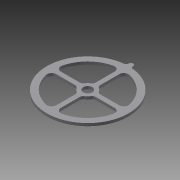
# Autodesk Inventor part: Vertical Thruster Grill 25090213
Saved by Autodesk Inventor 2013 (Build 170138000, 138)
## iProperties
Created: 2012-05-09
Part Number: Vertical Thruster Grill 25090213
Material: Generic
Document SubType Name: Modeling
Designer: user
Density: 1 g/cm^3
Author: user
Autodesk Inventor part; units mm, degrees
ref_plane "YZ Plane" through (0, 0, 0) normal (1, 0, 0) x (0, 1, 0)
ref_plane "XZ Plane" through (0, 0, 0) normal (0, 1, 0) x (-1, 0, 0)
ref_plane "XY Plane" through (0, 0, 0) normal (0, 0, 1) x (1, 0, 0)
sketch "Sketch1" plane through (0, 0, 0) normal (0, 0, 1) x (1, 0, 0)
  arc A0 (-4.7368, 44.75) -> (4.7368, 44.75) centre (0, 0) ccw
  line L0 (-32.2391, 2.5) -> (-11.2583, 2.5)
  line L1 (11.2583, 2.5) -> (32.2391, 2.5)
  line L2 (-2.5, 32.2391) -> (-2.5, 11.2583)
  line L3 (-2.5, -11.2583) -> (-2.5, -32.2391)
  line L4 (-32.2391, -2.5) -> (-11.2583, -2.5)
  line L5 (11.2583, -2.5) -> (32.2391, -2.5)
  line L6 (2.5, 32.2391) -> (2.5, 11.2583)
  line L7 (2.5, -11.2583) -> (2.5, -32.2391)
  arc A1 (-8.6329, 37.1091) -> (-37.1091, 8.6329) centre (0, 0) ccw
  arc A2 (37.1091, 8.6329) -> (8.6329, 37.1091) centre (0, 0) ccw
  arc A3 (-37.1091, -8.6329) -> (-8.6329, -37.1091) centre (0, 0) ccw
  arc A4 (8.6329, -37.1091) -> (37.1091, -8.6329) centre (0, 0) ccw
  arc A5 (-2.5, 32.2391) -> (-8.6329, 37.1091) centre (-7.5, 32.2391) ccw
  arc A6 (8.6329, 37.1091) -> (2.5, 32.2391) centre (7.5, 32.2391) ccw
  arc A7 (32.2391, 2.5) -> (37.1091, 8.6329) centre (32.2391, 7.5) ccw
  arc A8 (37.1091, -8.6329) -> (32.2391, -2.5) centre (32.2391, -7.5) ccw
  arc A9 (2.5, -32.2391) -> (8.6329, -37.1091) centre (7.5, -32.2391) ccw
  arc A10 (-8.6329, -37.1091) -> (-2.5, -32.2391) centre (-7.5, -32.2391) ccw
  arc A11 (-32.2391, -2.5) -> (-37.1091, -8.6329) centre (-32.2391, -7.5) ccw
  arc A12 (-37.1091, 8.6329) -> (-32.2391, 2.5) centre (-32.2391, 7.5) ccw
  line L8 (-2.5, 47.2361) -> (-2.5, 47.5)
  line L9 (0, 50) -> (0, 50)
  line L10 (2.5, 47.5) -> (2.5, 47.2361)
  arc A13 (0, 50) -> (-2.5, 47.5) centre (0, 47.5) ccw
  arc A14 (2.5, 47.5) -> (0, 50) centre (0, 47.5) ccw
  arc A15 (2.5, 47.2361) -> (4.7368, 44.75) centre (5, 47.2361) ccw
  arc A16 (-4.7368, 44.75) -> (-2.5, 47.2361) centre (-5, 47.2361) ccw
  circle A17 centre (0, 0) radius 5
  arc A18 (-4.5, 7.7942) -> (-7.7942, 4.5) centre (0, 0) ccw
  arc A19 (7.7942, 4.5) -> (4.5, 7.7942) centre (0, 0) ccw
  arc A20 (-7.7942, -4.5) -> (-4.5, -7.7942) centre (0, 0) ccw
  arc A21 (4.5, -7.7942) -> (7.7942, -4.5) centre (0, 0) ccw
  arc A22 (-11.2583, 2.5) -> (-7.7942, 4.5) centre (-11.2583, 6.5) ccw
  arc A23 (-4.5, 7.7942) -> (-2.5, 11.2583) centre (-6.5, 11.2583) ccw
  arc A24 (2.5, 11.2583) -> (4.5, 7.7942) centre (6.5, 11.2583) ccw
  arc A25 (7.7942, 4.5) -> (11.2583, 2.5) centre (11.2583, 6.5) ccw
  arc A26 (11.2583, -2.5) -> (7.7942, -4.5) centre (11.2583, -6.5) ccw
  arc A27 (4.5, -7.7942) -> (2.5, -11.2583) centre (6.5, -11.2583) ccw
  arc A28 (-2.5, -11.2583) -> (-4.5, -7.7942) centre (-6.5, -11.2583) ccw
  arc A29 (-7.7942, -4.5) -> (-11.2583, -2.5) centre (-11.2583, -6.5) ccw
  point P0 (-2.5, 38.0179)
  point P1 (2.5, 38.0179)
  point P2 (-38.0179, -2.5)
  point P3 (-38.0179, 2.5)
  point P4 (38.0179, -2.5)
  point P5 (38.0179, 2.5)
  point P6 (2.5, -38.0179)
  point P7 (-2.5, -38.0179)
  point P8 (-2.5, 44.9305)
  point P9 (2.5, 44.9305)
  point P10 (-2.5, 8.6458)
  point P11 (2.5, 8.6458)
  point P12 (8.6458, 2.5)
  point P13 (8.6458, -2.5)
  point P14 (2.5, -8.6458)
  point P15 (-2.5, -8.6458)
  point P16 (-8.6458, -2.5)
  point P17 (-8.6458, 2.5)
  dimension "d0" = 90
  dimension "d7" = 2.5
  dimension "d8" = 2.5
  dimension "d9" = 2.5
  dimension "d10" = 5
  dimension "d11" = 5
  dimension "d12" = 5
  dimension "d13" = 5
  dimension "d14" = 38.1
  dimension "d15" = 38.1
  dimension "d16" = 38.1
  dimension "d17" = 38.1
  dimension "d18" = 5
  dimension "d19" = 5
  dimension "d20" = 50
  dimension "d21" = 2.5
  dimension "d24" = 10
  dimension "d27" = 4
  constraints: 76 point on circle, 40 tangent, 30 centre point, 22 end point, 19 point on line, 17 equal radius, 10 parallel, 5 perpendicular, 4 coincident
  measures "d0" diameter of A0
  measures "d7" distance from line of L1 point (0, 0)
  measures "d8" distance from line of L7 point (0, 0)
  measures "d9" distance from line of L0 point (0, 0)
  measures "d10" distance between parallel lines of L6 L2
  measures "d11" distance between parallel lines of L5 L1
  measures "d12" distance between parallel lines of L7 L3
  measures "d13" distance between parallel lines of L0 L4
  measures "d14" radius of A1
  measures "d15" radius of A2
  measures "d16" radius of A4
  measures "d17" radius of A3
  measures "d18" radius of A5
  measures "d19" distance between parallel lines of L8 L10
  measures "d20" distance from line of point (0, 0) L9
  measures "d21" radius of A13
  measures "d24" diameter of A17
  measures "d27" radius of A22
extrude "Extrusion2" add sketch "Sketch1" along normal blind 3
body "Solid2"
